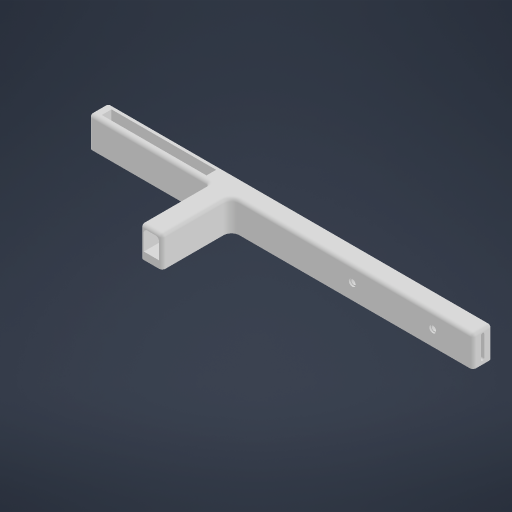
# Autodesk Inventor part: Rod
Saved by Autodesk Inventor 2024.1 (Build 281209000, 209)
## iProperties
Created: 2023-09-06
Part Number: Rod
Material: Generic
Document SubType Name: Modeling
Designer: User
Density: 1 g/cm^3
Appearance: Default
Author: User
Autodesk Inventor part; units mm, degrees
ref_plane "YZ Plane" through (0, 0, 0) normal (1, 0, 0) x (0, 1, 0)
ref_plane "XZ Plane" through (0, 0, 0) normal (0, 1, 0) x (-1, 0, 0)
ref_plane "XY Plane" through (0, 0, 0) normal (0, 0, 1) x (1, 0, 0)
sketch "Sketch1" plane through (0, 0, 0) normal (0, 0, 1) x (1, 0, 0)
  line L0 (0, 0) -> (-13.5, 0)
  line L1 (-13.5, 0) -> (-13.5, 19)
  line L2 (-13.5, 19) -> (0, 19)
  line L3 (0, 19) -> (0, 0)
  dimension "d0" = 13.5
  dimension "d1" = 19
  constraints: 8 end point, 2 parallel, 1 horizontal, 1 perpendicular
  measures "d0" distance of L1.end L2.end
  measures "d1" distance of L0.end L1.end
extrude "Extrusion1" add sketch "Sketch1" along normal blind 15 and the other way blind 40
sketch "Sketch2" plane through (0, 0, 15) normal (0, 0, 1) x (1, 0, 0)
  line L0 (-13.5, 19) -> (-13.5, 0) projected
  line L1 (-13.5, 0) -> (-11.45, 0)
  line L2 (-11.45, 0) -> (-11.45, 4.55)
  line L3 (-11.45, 4.55) -> (-13.5, 4.55)
  line L4 (-13.5, 4.55) -> (-13.5, 0)
  line L5 (0, 19) -> (-13.5, 19) projected
  line L6 (0, 19) -> (-2.05, 19)
  line L7 (-2.05, 19) -> (-2.05, 16.95)
  line L8 (-2.05, 16.95) -> (0, 16.95)
  line L9 (0, 16.95) -> (0, 19)
  line L10 (-11.45, 4.55) -> (-2.05, 4.55)
  line L11 (-2.05, 4.55) -> (-2.05, 16.95)
  line L12 (-2.05, 16.95) -> (-11.45, 16.95)
  line L13 (-11.45, 16.95) -> (-11.45, 4.55)
  point P0 (0, 0)
  dimension "d4" = 2.05
  dimension "d5" = 4.55
  dimension "d6" = 2.05
  dimension "d7" = 2.05
  constraints: 24 end point, 6 parallel, 3 horizontal, 3 perpendicular
  measures "d4" distance of L3.end L2.end
  measures "d5" distance of L2.end L1.end
  measures "d6" distance of L8.end L7.end
  measures "d7" distance of L7.end L6.end
extrude "Extrusion2" cut sketch "Sketch2" against normal blind 50 contours L13 L12 L11 L10
fillet "Fillet9" radius 2 2 edges at (-2.05, 16.95, -10) (-11.45, 16.95, -10)
sketch "Sketch5" plane through (0, 0, 15) normal (1, 0, 0) x (0, 0, -1)
  line L0 (55, 19) -> (0, 19) projected
  line L1 (55, 19) -> (43, 19)
  line L2 (43, 19) -> (43, 0)
  line L3 (43, 0) -> (55, 0)
  line L4 (55, 0) -> (55, 19)
  point P0 (15, 0)
  dimension "d14" = 12
  dimension "d15" = 19
  constraints: 8 end point, 2 parallel, 1 horizontal, 1 perpendicular
  measures "d14" distance of L3.end L2.end
  measures "d15" distance of L2.end L1.end
extrude "Extrusion3" add sketch "Sketch5" along normal blind 150
sketch "Sketch7" plane through (0, 0, -28) normal (0, 0, 1) x (1, 0, 0)
  line L0 (0, 19) -> (150, 19) projected
  line L1 (25, 19) -> (34.5, 19) construction
  line L2 (0, 0) -> (150, 0) projected
  line L3 (25, 0) -> (34.5, 0) construction
  point P0 (125, 9.5)
  point P1 (75, 9.5)
  constraints: 4 end point, 2 horizontal, 2 point on line
hole "Hole1" at (75, 9.5, -28) at (125, 9.5, -28) direction (0, 0, -1) diameter 3.2 depth 7 counterbore diameter 4.2 counterbore depth 1
sketch "Sketch10" plane through (150, 0, 15) normal (1, 0, 0) x (0, 0, -1)
  line L0 (55, 0) -> (50, 0)
  line L1 (50, 0) -> (50, 2)
  line L2 (50, 2) -> (55, 2)
  line L3 (55, 2) -> (55, 0)
  line L4 (50, 2) -> (48, 2)
  line L5 (48, 2) -> (48, 17)
  line L6 (48, 17) -> (50, 17)
  line L7 (50, 17) -> (50, 2)
  point P0 (15, 0)
  dimension "d46" = 5
  dimension "d47" = 2
  dimension "d48" = 2
  dimension "d49" = 15
  constraints: 16 end point, 4 parallel, 2 horizontal, 2 perpendicular
  measures "d46" distance of L1.end L2.end
  measures "d47" distance of L0.end L1.end
  measures "d48" distance of L5.end L6.end
  measures "d49" distance of L4.end L5.end
extrude "Extrusion6" cut sketch "Sketch10" against normal blind 100 contours L4 L5 L6 L7
fillet "Fillet6" radius 5 1 edges at (0, 9.5, -28)
fillet "Fillet10" radius 1 4 edges at (100, 2, -35) (100, 2, -33) (100, 17, -35) (100, 17, -33)
sketch "Sketch13" plane through (-13.5, 0, 15) normal (-1, 0, 0) x (0, 0, 1)
  line L0 (-54.9881, 18.9995) -> (-42.9881, 18.9995)
  line L1 (-42.9881, 18.9995) -> (-42.9881, -0.0005)
  line L2 (-42.9881, -0.0005) -> (-54.9881, -0.0005)
  line L3 (-54.9881, -0.0005) -> (-54.9881, 18.9995)
  point P0 (-15, 0)
  dimension "d66" = 12
  dimension "d67" = 19
  constraints: 8 end point, 2 parallel, 1 horizontal, 1 perpendicular, 1 other
  measures "d66" distance of L1.end L2.end
  measures "d67" distance of L0.end L1.end
extrude "Extrusion8" add sketch "Sketch13" along normal blind 75
sketch "Sketch14" plane through (-13.5, 18.9995, -27.9881) normal (0, 1, 0) x (1, 0, 0)
  line L0 (-75, 12) -> (-75, 0) projected
  line L1 (-75, 12) -> (-70, 12)
  line L2 (-70, 12) -> (-70, 9)
  line L3 (-70, 9) -> (-75, 9)
  line L4 (-75, 9) -> (-75, 12)
  line L5 (0, 12.0119) -> (0, -42.9881) projected
  line L6 (0, 0) -> (-5, 0)
  line L7 (-5, 0) -> (-5, 3)
  line L8 (-5, 3) -> (0, 3)
  line L9 (0, 3) -> (0, 0)
  line L10 (-5, 3) -> (-70, 3)
  line L11 (-70, 3) -> (-70, 9)
  line L12 (-70, 9) -> (-5, 9)
  line L13 (-5, 9) -> (-5, 3)
  point P0 (13.5, -27.9881)
  dimension "d70" = 5
  dimension "d71" = 3
  dimension "d72" = 5
  dimension "d73" = 3
  constraints: 24 end point, 6 parallel, 3 horizontal, 3 perpendicular, 1 point on line
  measures "d70" distance of L2.end L3.end
  measures "d71" distance of L1.end L2.end
  measures "d72" distance of L7.end L8.end
  measures "d73" distance of L6.end L7.end
extrude "Extrusion9" cut sketch "Sketch14" against normal blind 14 contours L12 L13 L10 L11
fillet "Fillet11" radius 2 17 edges at (1.4645, 19, -26.5355) (77.5, 19, -28) (150, 9.5, -28) (0, 19, -4) (150, 9.5, -40) (68.25, 19, -40) (-51, 18.9995, -39.9881) (-13.5, 9.4997, -27.9881) (-51, 18.9995, -27.9881) (-13.5, 19, -12.5) (-88.5, 9.4995, -27.9881) (-88.5, 9.4995, -39.9881) (-13.5, 9.5, 15) (0, 9.5, 15) (-88.5, 18.9995, -33.9881) (-6.75, 19, 15) (150, 19, -34)
body "Solid1"
